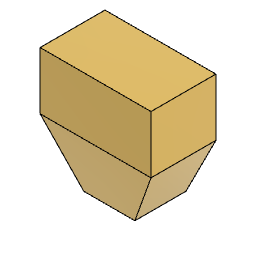
upper_single_connector (Autodesk Fusion 360 design; units mm, degrees)
Autodesk Fusion 360 part; units mm, degrees
sketch "Sketch1" plane through (0, 0, 0) normal (0, 1, 0) x (1, 0, 0)
  line L0 (7.9, 2.9) -> (7.9, 4.9)
  line L1 (-2.7515, -3.6) -> (-4.9, -5.7485)
  line L2 (2.9, -7.9) -> (4.9, -7.9)
  line L3 (-2.9, -7.9) -> (-2.9, -10.1)
  arc A0 (-10.1, -9) -> (-9, -10.1) centre (-9, -9) ccw
  line L4 (5.7485, 4.9) -> (3.6, 2.7515)
  line L5 (-7.9, 2.9) -> (-10.1, 2.9)
  line L6 (-4.9, -7.9) -> (-2.9, -7.9)
  line L7 (4.9, 5.7485) -> (4.9, 7.9)
  line L8 (10.1, 2.9) -> (7.9, 2.9)
  line L9 (9, -10.1) -> (2.9, -10.1)
  arc A1 (9, -10.1) -> (10.1, -9) centre (9, -9) ccw
  line L10 (4.9, -5.7485) -> (2.7515, -3.6)
  line L11 (5.7485, -4.9) -> (7.9, -4.9)
  line L12 (-10.1, 2.9) -> (-10.1, 9)
  line L13 (7.9, -2.9) -> (10.1, -2.9)
  line L14 (-3.6, 2.7515) -> (-5.7485, 4.9)
  line L15 (10.1, -2.9) -> (10.1, -9)
  line L16 (-2.9, 10.1) -> (-2.9, 7.9)
  line L17 (7.9, -4.9) -> (7.9, -2.9)
  line L18 (-3.6, -2.7515) -> (-3.6, 2.7515)
  line L19 (3.6, 2.7515) -> (3.6, -2.7515)
  line L20 (2.7515, -3.6) -> (-2.7515, -3.6)
  line L21 (-10.1, -9) -> (-10.1, -2.9)
  line L22 (10.1, 9) -> (10.1, 2.9)
  line L23 (2.9, 7.9) -> (2.9, 10.1)
  line L24 (7.9, 4.9) -> (5.7485, 4.9)
  line L25 (-2.9, -10.1) -> (-9, -10.1)
  line L26 (-2.7515, 3.6) -> (2.7515, 3.6)
  arc A2 (-9, 10.1) -> (-10.1, 9) centre (-9, 9) ccw
  line L27 (4.9, 7.9) -> (2.9, 7.9)
  line L28 (-7.9, -4.9) -> (-5.7485, -4.9)
  line L29 (2.9, 10.1) -> (9, 10.1)
  arc A3 (10.1, 9) -> (9, 10.1) centre (9, 9) ccw
  line L30 (-4.9, -5.7485) -> (-4.9, -7.9)
  line L31 (-7.9, -2.9) -> (-7.9, -4.9)
  line L32 (-4.9, 7.9) -> (-4.9, 5.7485)
  line L33 (2.7515, 3.6) -> (4.9, 5.7485)
  line L34 (-4.9, 5.7485) -> (-2.7515, 3.6)
  line L35 (-10.1, -2.9) -> (-7.9, -2.9)
  line L36 (3.6, -2.7515) -> (5.7485, -4.9)
  line L37 (4.9, -7.9) -> (4.9, -5.7485)
  line L38 (2.9, -10.1) -> (2.9, -7.9)
  line L39 (-5.7485, -4.9) -> (-3.6, -2.7515)
  line L40 (-7.9, 4.9) -> (-7.9, 2.9)
  line L41 (-2.9, 7.9) -> (-4.9, 7.9)
  line L42 (-9, 10.1) -> (-2.9, 10.1)
  line L43 (-5.7485, 4.9) -> (-7.9, 4.9)
  line L44 (-15.1, -14.6) -> (13.1, -14.6)
  line L45 (13.1, -14.6) -> (13.1, 14.6)
  line L46 (13.1, 14.6) -> (-15.1, 14.6)
  line L47 (-15.1, 14.6) -> (-15.1, -14.6)
  dimension "d1" = 3
  dimension "d2" = 5
  dimension "d3" = 4.5
  dimension "d4" = 4.5
  constraint horizontal L44
  constraint vertical L45
  constraint horizontal L46
  constraint vertical L47
  measures "d1" distance of L15 L45
  measures "d2" distance of L21 L47
  measures "d3" distance of L9 L44
  measures "d4" distance of L29 L46
extrude "Extrude1" add sketch "Sketch1" along normal blind 3 contours L0 L1 L2 L3 A0 L4 L5 L6 L7 L8 L9 A1 L10 L11 L12 L13 L14 L15 L16 L17 L18 L19 L20 L21 L22 L23 L24 L25 L26 A2 L27 L28 L29 A3 L30 L31 L32 L33 L34 L35 L36 L37 L38 L39 L40 L41 L42 L43 | L44 L45 L46 L47
extrude "Extrude2" add sketch "Sketch1" along normal blind 30 from surface at 3
mirror "Mirror1" about plane through (-15.1, 0, -14.6) normal (-1, 0, 0) of bodies 1 merged
ref_plane "WorkPlane1" through (-15.1, 16.5, -44.6) normal (0, 0, -1) x (-1, 0, 0)
sketch "Sketch2" plane through (0, 0, -44.6) normal (0, 0, -1) x (-1, 0, 0)
  line L0 (-13.1, 0) -> (43.3, 0)
  line L1 (43.3, 0) -> (43.3, 33)
  line L2 (43.3, 33) -> (-13.1, 33)
  line L3 (-13.1, 33) -> (-13.1, 0)
  line L4 (28.1, 33) -> (2.1, 33)
  line L5 (2.1, 33) -> (2.1, 7)
  line L6 (2.1, 7) -> (28.1, 7)
  line L7 (28.1, 7) -> (28.1, 33)
  line L8 (15.1, 33) -> (15.1, 0) construction
  line L9 (25.3, 30.2) -> (4.9, 30.2)
  line L10 (4.9, 30.2) -> (4.9, 9.8)
  line L11 (4.9, 9.8) -> (25.3, 9.8)
  line L12 (25.3, 9.8) -> (25.3, 30.2)
  dimension "d15" = 20.4
  dimension "d17" = 2.8
  dimension "d18" = 2.8
  dimension "d29" = 2.8
  constraint horizontal L4
  constraint vertical L5
  constraint horizontal L6
  constraint vertical L7
  constraint coincident L2 L4.start
  constraint coincident L2 L8.start
  constraint coincident L0 L8.end
  constraint perpendicular L0 L8
  constraint midpoint L0 L8.end
  constraint symmetric L5 L7 L8
  constraint horizontal L9
  constraint vertical L10
  constraint horizontal L11
  constraint vertical L12
  constraint equal L5 L6
  constraint equal L10 L11
  measures "d15" distance of L10.end L11.end
  measures "d17" horizontal distance of L6.end L11.end
  measures "d18" horizontal distance of L5.end L10.end
  measures "d29" distance of L6 L11
loft "Loft1" add profiles "Sketch2" section 1 face at (-5.7, 11, -14.6) section 2 contours L2 L4 L5 L6 L7 | L9 L10 L11 L12
extrude "Extrude3" cut sketch "Sketch2" against normal blind 30 contours L9 L10 L11 L12
sketch "Sketch3" plane through (0, 33, 0) normal (0, 1, 0) x (-1, 0, 0)
  line L0 (21.2, 10.1) -> (27.3, 10.1)
  line L1 (27.3, 10.1) -> (27.3, 7.9)
  line L2 (27.3, 7.9) -> (25.3, 7.9)
  line L3 (25.3, 7.9) -> (25.3, 5.7485)
  line L4 (25.3, 5.7485) -> (27.4485, 3.6)
  line L5 (27.4485, 3.6) -> (32.9515, 3.6)
  line L6 (32.9515, 3.6) -> (35.1, 5.7485)
  line L7 (35.1, 5.7485) -> (35.1, 7.9)
  line L8 (35.1, 7.9) -> (33.1, 7.9)
  line L9 (33.1, 7.9) -> (33.1, 10.1)
  line L10 (33.1, 10.1) -> (39.2, 10.1)
  arc A0 (40.3, 9) -> (39.2, 10.1) centre (39.2, 9) ccw
  line L11 (40.3, 9) -> (40.3, 2.9)
  line L12 (40.3, 2.9) -> (38.1, 2.9)
  line L13 (38.1, 2.9) -> (38.1, 4.9)
  line L14 (38.1, 4.9) -> (35.9485, 4.9)
  line L15 (35.9485, 4.9) -> (33.8, 2.7515)
  line L16 (33.8, 2.7515) -> (33.8, -2.7515)
  line L17 (33.8, -2.7515) -> (35.9485, -4.9)
  line L18 (35.9485, -4.9) -> (38.1, -4.9)
  line L19 (38.1, -4.9) -> (38.1, -2.9)
  line L20 (38.1, -2.9) -> (40.3, -2.9)
  line L21 (40.3, -2.9) -> (40.3, -9)
  arc A1 (39.2, -10.1) -> (40.3, -9) centre (39.2, -9) ccw
  line L22 (39.2, -10.1) -> (33.1, -10.1)
  line L23 (33.1, -10.1) -> (33.1, -7.9)
  line L24 (33.1, -7.9) -> (35.1, -7.9)
  line L25 (35.1, -7.9) -> (35.1, -5.7485)
  line L26 (35.1, -5.7485) -> (32.9515, -3.6)
  line L27 (32.9515, -3.6) -> (27.4485, -3.6)
  line L28 (27.4485, -3.6) -> (25.3, -5.7485)
  line L29 (25.3, -5.7485) -> (25.3, -7.9)
  line L30 (25.3, -7.9) -> (27.3, -7.9)
  line L31 (27.3, -7.9) -> (27.3, -10.1)
  line L32 (27.3, -10.1) -> (21.2, -10.1)
  arc A2 (20.1, -9) -> (21.2, -10.1) centre (21.2, -9) ccw
  line L33 (20.1, -9) -> (20.1, -2.9)
  line L34 (20.1, -2.9) -> (22.3, -2.9)
  line L35 (22.3, -2.9) -> (22.3, -4.9)
  line L36 (22.3, -4.9) -> (24.4515, -4.9)
  line L37 (24.4515, -4.9) -> (26.6, -2.7515)
  line L38 (26.6, -2.7515) -> (26.6, 2.7515)
  line L39 (26.6, 2.7515) -> (24.4515, 4.9)
  line L40 (24.4515, 4.9) -> (22.3, 4.9)
  line L41 (22.3, 4.9) -> (22.3, 2.9)
  line L42 (22.3, 2.9) -> (20.1, 2.9)
  line L43 (20.1, 2.9) -> (20.1, 9)
  arc A3 (21.2, 10.1) -> (20.1, 9) centre (21.2, 9) ccw
  line L44 (2.9, 10.1) -> (9, 10.1)
  arc A4 (10.1, 9) -> (9, 10.1) centre (9, 9) ccw
  line L45 (10.1, 9) -> (10.1, 2.9)
  line L46 (10.1, 2.9) -> (7.9, 2.9)
  line L47 (7.9, 2.9) -> (7.9, 4.9)
  line L48 (7.9, 4.9) -> (5.7485, 4.9)
  line L49 (5.7485, 4.9) -> (3.6, 2.7515)
  line L50 (3.6, 2.7515) -> (3.6, -2.7515)
  line L51 (3.6, -2.7515) -> (5.7485, -4.9)
  line L52 (5.7485, -4.9) -> (7.9, -4.9)
  line L53 (7.9, -4.9) -> (7.9, -2.9)
  line L54 (7.9, -2.9) -> (10.1, -2.9)
  line L55 (10.1, -2.9) -> (10.1, -9)
  arc A5 (9, -10.1) -> (10.1, -9) centre (9, -9) ccw
  line L56 (9, -10.1) -> (2.9, -10.1)
  line L57 (2.9, -10.1) -> (2.9, -7.9)
  line L58 (2.9, -7.9) -> (4.9, -7.9)
  line L59 (4.9, -7.9) -> (4.9, -5.7485)
  line L60 (4.9, -5.7485) -> (2.7515, -3.6)
  line L61 (2.7515, -3.6) -> (-2.7515, -3.6)
  line L62 (-2.7515, -3.6) -> (-4.9, -5.7485)
  line L63 (-4.9, -5.7485) -> (-4.9, -7.9)
  line L64 (-4.9, -7.9) -> (-2.9, -7.9)
  line L65 (-2.9, -7.9) -> (-2.9, -10.1)
  line L66 (-2.9, -10.1) -> (-9, -10.1)
  arc A6 (-10.1, -9) -> (-9, -10.1) centre (-9, -9) ccw
  line L67 (-10.1, -9) -> (-10.1, -2.9)
  line L68 (-10.1, -2.9) -> (-7.9, -2.9)
  line L69 (-7.9, -2.9) -> (-7.9, -4.9)
  line L70 (-7.9, -4.9) -> (-5.7485, -4.9)
  line L71 (-5.7485, -4.9) -> (-3.6, -2.7515)
  line L72 (-3.6, -2.7515) -> (-3.6, 2.7515)
  line L73 (-3.6, 2.7515) -> (-5.7485, 4.9)
  line L74 (-5.7485, 4.9) -> (-7.9, 4.9)
  line L75 (-7.9, 4.9) -> (-7.9, 2.9)
  line L76 (-7.9, 2.9) -> (-10.1, 2.9)
  line L77 (-10.1, 2.9) -> (-10.1, 9)
  arc A7 (-9, 10.1) -> (-10.1, 9) centre (-9, 9) ccw
  line L78 (-9, 10.1) -> (-2.9, 10.1)
  line L79 (-2.9, 10.1) -> (-2.9, 7.9)
  line L80 (-2.9, 7.9) -> (-4.9, 7.9)
  line L81 (-4.9, 7.9) -> (-4.9, 5.7485)
  line L82 (-4.9, 5.7485) -> (-2.7515, 3.6)
  line L83 (-2.7515, 3.6) -> (2.7515, 3.6)
  line L84 (2.7515, 3.6) -> (4.9, 5.7485)
  line L85 (4.9, 5.7485) -> (4.9, 7.9)
  line L86 (4.9, 7.9) -> (2.9, 7.9)
  line L87 (2.9, 7.9) -> (2.9, 10.1)
  line L88 (43.3, -14.6) -> (43.3, 14.6)
  line L89 (43.3, 14.6) -> (-13.1, 14.6)
  line L90 (-13.1, 14.6) -> (-13.1, -14.6)
  line L91 (-13.1, -14.6) -> (2.1, -44.6)
  line L92 (2.1, -44.6) -> (28.1, -44.6)
  line L93 (28.1, -44.6) -> (43.3, -14.6)
  line L94 (15.1, -44.6) -> (15.1, -17.6132) construction
  circle A8 centre (15.1, -37.1) radius 2
  circle A9 centre (15.1, -22.1) radius 2
  dimension "d23" = 4
  dimension "d24" = 7.5
  dimension "d25" = 15
  constraint midpoint L92 L94.start
  constraint perpendicular L92 L94
  constraint coincident L94 A8.centre
  constraint coincident L94 A9.centre
  constraint equal A8 A9
  measures "d23" diameter of A8
  measures "d24" distance of L94.start A8.centre
  measures "d25" distance of A8.centre A9.centre
extrude "Extrude4" cut sketch "Sketch3" against normal blind 4 contours A8 | A9
equation "d15 = 20 mm + 2 * gap"
equation "d17 = 3 mm - gap"
equation "d18 = 3 mm - gap"
equation "gap = 0.2 mm"
equation "d29 = 3 mm - gap"
